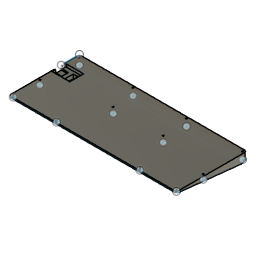
RowLow52V2-bottomcase v4 (Autodesk Fusion 360 design; units mm, degrees)
Autodesk Fusion 360 part; units mm, degrees
sketch "スケッチ1" plane through (0, 0, 0) normal (0, 0, 1) x (1, 0, 0)
  line L0 (239.1777, -2.4183) -> (239.1601, -97.857)
  spline S0 degree 3 poles (239.1601, -97.857) (239.1855, -99.2018) (238.1172, -100.3131) (236.7725, -100.3413) knots 0 0 0 0 1 1 1 1
  line L1 (236.7725, -100.3413) -> (2.6363, -100.3547)
  spline S1 degree 3 poles (2.6363, -100.3547) (1.2915, -100.3801) (0.1799, -99.3119) (0.152, -97.9671) knots 0 0 0 0 1 1 1 1
  line L2 (0.152, -97.9671) -> (0.152, -2.5093)
  spline S2 degree 3 poles (0.152, -2.5093) (0.1266, -1.1645) (1.1949, -0.0529) (2.5393, -0.025) knots 0 0 0 0 1 1 1 1
  line L3 (2.5393, -0.025) -> (236.6931, -0.031)
  spline S3 degree 3 poles (236.6931, -0.031) (238.0382, -0.0053) (239.1498, -1.0739) (239.1777, -2.4183) knots 0 0 0 0 1 1 1 1
  line L4 (1.676, -20.726) -> (1.676, -20.98)
  line L5 (1.676, -20.98) -> (1.676, -40.4107)
  line L6 (1.676, -40.4107) -> (26.695, -40.4107)
  line L7 (26.695, -40.4107) -> (26.695, -20.7257)
  line L8 (26.695, -20.7257) -> (2.311, -20.7257)
  line L9 (2.311, -20.7257) -> (1.676, -20.726)
  line L10 (1.676, -20.726) -> (1.676, -20.98)
  line L11 (10.312, -35.204) -> (10.312, -35.458)
  line L12 (2.692, -26.06) -> (0.025, -26.06)
  line L13 (0.025, -26.06) -> (0.025, -35.458)
  line L14 (0.025, -35.458) -> (10.312, -35.458)
  line L15 (10.312, -35.458) -> (10.312, -35.204)
  line L16 (10.312, -35.204) -> (10.312, -26.06)
  line L17 (10.312, -26.06) -> (2.692, -26.06)
  line L18 (22.123, -37.236) -> (22.123, -24.282)
  line L19 (22.123, -24.282) -> (15.646, -24.282)
  line L20 (15.646, -24.282) -> (15.646, -37.236)
  line L21 (15.646, -37.236) -> (22.123, -37.236)
  circle A0 centre (155.346, -2.311) radius 1.1
  circle A1 centre (236.2447, -3.073) radius 1.1
  circle A2 centre (183.921, -97.561) radius 1.1
  circle A3 centre (2.946, -97.561) radius 1.1
  circle A4 centre (2.946, -59.461) radius 1.1
  circle A5 centre (88.798, -40.411) radius 1.1
  circle A6 centre (64.922, -97.561) radius 1.1
  circle A7 centre (160.172, -40.411) radius 1.1
  circle A8 centre (79.273, -2.565) radius 1.1
  circle A9 centre (236.372, -59.461) radius 1.1
  circle A10 centre (236.2447, -97.561) radius 1.1
  circle A11 centre (2.946, -2.819) radius 1.1
  point P0 (156.446, -2.311)
  point P1 (237.3447, -3.073)
  point P2 (185.021, -97.561)
  point P3 (4.046, -97.561)
  point P4 (4.046, -59.461)
  point P5 (89.898, -40.411)
  point P6 (66.022, -97.561)
  point P7 (161.272, -40.411)
  point P8 (80.373, -2.565)
  point P9 (237.472, -59.461)
  point P10 (237.3447, -97.561)
  point P11 (4.046, -2.819)
extrude "押し出し1" add sketch "スケッチ1" against normal blind 40 contours L0 S0 L1 S1 L2 S2 L3 S3 L4 L5 L6 L7 L8 L9 L10 L12 L14 | L2 L5 L12 L14 | L5 L11 L12 L14 L15 L16 L17 | L4 L5 L6 L7 L8 L9 L10 L11 L12 L14 L15 L16 L17 | L18 L19 L20 L21
extrude "押し出し2" cut sketch "スケッチ1" against normal blind 6 contours L2 L5 L12 L14 | L5 L11 L12 L14 L15 L16 L17
extrude "押し出し3" cut sketch "スケッチ1" against normal blind 4 contours L4 L5 L6 L7 L8 L9 L10 L11 L12 L14 L15 L16 L17
extrude "押し出し4" cut sketch "スケッチ1" against normal blind 40 contours L18 L19 L20 L21
sketch "スケッチ2" plane through (0, 0, 0) normal (1, 0, 0) x (0, 1, 0)
  line L0 (-100.355, 0) -> (-100.355, -2)
  line L1 (-100.355, -2) -> (3, -13)
  line L2 (-7.5019, -11.8823) -> (0.5, -9)
  line L3 (-100.355, -2) -> (-100.57, -2)
  line L4 (-100.57, -2) -> (-100.57, -3.4)
  line L5 (-100.57, -3.4) -> (-100.57, -40.4093)
  line L6 (-100.57, -40.4093) -> (-74, -40.4093)
  line L7 (-74, -40.4093) -> (1, -40.4093)
  line L8 (1, -40.4093) -> (0.5, -9)
  dimension "d9" = 2
  constraint vertical L0
  constraint coincident L1 L2.start
  constraint perpendicular L0 L3
  constraint perpendicular L3 L4
  constraint parallel L4 L5
  constraint perpendicular L5 L6
  constraint parallel L6 L7
  measures "d9" distance of L0.start L0.end
extrude "押し出し5" cut sketch "スケッチ2" along normal blind 400 contours L1 L3 L4 L5 L6 L7 L8
extrude "押し出し6" cut sketch "スケッチ2" along normal blind 400 contours L1 L2 L8
sketch "スケッチ3" plane through (0, 0, 0) normal (1, 0, 0) x (0, 1, 0)
  line L0 (0.1398, 0.1029) -> (-26.06, 0.1029)
  constraint horizontal L0
sketch "スケッチ4" plane through (0, -1.3345, -12.5387) normal (0, -0.105832, -0.994384) x (1, 0, 0)
  ellipse E0 centre (160.172, 39.2973) end of major axis (160.172, 38.1911) minor radius 1.1
  ellipse E1 centre (236.2447, 96.77) end of major axis (236.2447, 95.6638) minor radius 1.1
  ellipse E2 centre (183.921, 96.77) end of major axis (183.921, 95.6638) minor radius 1.1
  ellipse E3 centre (236.372, 58.4548) end of major axis (236.372, 57.3487) minor radius 1.1
  ellipse E4 centre (88.798, 39.2973) end of major axis (88.798, 38.1911) minor radius 1.1
  ellipse E5 centre (2.946, 96.77) end of major axis (2.946, 95.6638) minor radius 1.1
  ellipse E6 centre (2.946, 58.4548) end of major axis (2.946, 57.3487) minor radius 1.1
  ellipse E7 centre (64.922, 96.77) end of major axis (64.922, 95.6638) minor radius 1.1
  line L0 (22.123, 36.1043) -> (22.123, 23.0772)
  line L1 (22.123, 23.0772) -> (15.646, 23.0772)
  line L2 (15.646, 23.0772) -> (15.646, 36.1043)
  line L3 (15.646, 36.1043) -> (22.123, 36.1043)
  line L4 (0.152, 6.2022) -> (239.1768, 6.2022)
  line L5 (239.1768, 6.2022) -> (239.1601, 97.0677)
  spline S0 degree 3 poles (236.7725, 99.566) (236.9396, 99.5624) (237.1056, 99.542) (237.4266, 99.4681) (237.5804, 99.4159) (238.0207, 99.2151) (238.2841, 99.0244) (238.7171, 98.5588) (238.8855, 98.2893) (239.1117, 97.6993) (239.166, 97.3855) (239.1601, 97.0677) knots -0.385662 -0.385662 -0.385662 -0.385662 -0.335417 -0.335417 -0.286659 -0.286659 -0.189937 -0.189937 -0.095378 -0.095378 0 0 0 0
  line L6 (236.7725, 99.566) -> (2.6363, 99.5794)
  spline S1 degree 3 poles (2.6151, 99.5798) (2.6222, 99.5797) (2.6292, 99.5796) (2.6363, 99.5794) knots -0.002119 -0.002119 -0.002119 -0.002119 0 0 0 0
  line L7 (2.6151, 99.5798) -> (2.5636, 99.5798)
  spline S2 degree 3 poles (0.152, 97.1784) (0.1556, 97.3498) (0.1766, 97.52) (0.2528, 97.8488) (0.3067, 98.0062) (0.5108, 98.4494) (0.702, 98.7126) (1.1661, 99.1426) (1.4326, 99.3091) (1.9922, 99.5233) (2.2757, 99.5767) (2.5636, 99.5798) knots -0.385525 -0.385525 -0.385525 -0.385525 -0.334027 -0.334027 -0.284114 -0.284114 -0.187392 -0.187392 -0.093864 -0.093864 -0.00728 -0.00728 -0.00728 -0.00728
  line L8 (0.152, 97.1784) -> (0.152, 6.2022)
  circle A0 centre (2.946, 96.77) radius 2.3941
  circle A1 centre (2.946, 58.4548) radius 2.3046
  circle A2 centre (64.922, 96.77) radius 2.3483
  circle A3 centre (183.921, 96.77) radius 2.2833
  circle A4 centre (236.2447, 96.77) radius 2.2651
  circle A5 centre (236.372, 58.4548) radius 2.3236
  circle A6 centre (160.172, 39.2973) radius 2.3586
  circle A7 centre (88.798, 39.2973) radius 2.4454
  constraint concentric E5 A0
  constraint concentric E6 A1
  constraint concentric E7 A2
  constraint concentric E2 A3
  constraint concentric E1 A4
  constraint concentric E3 A5
  constraint concentric E0 A6
  constraint concentric E4 A7
extrude "押し出し7" cut sketch "スケッチ4" against normal blind 1 contours E5 | A0
extrude "押し出し8" cut sketch "スケッチ4" against normal blind 1 contours E7 | A2
extrude "押し出し9" cut sketch "スケッチ4" against normal blind 1 contours E2 | A3
extrude "押し出し10" cut sketch "スケッチ4" against normal blind 1 contours E1 | A4
extrude "押し出し11" cut sketch "スケッチ4" against normal blind 1.5 contours E6 | A1
extrude "押し出し12" cut sketch "スケッチ4" against normal blind 1.5 contours E4 | A7
extrude "押し出し13" cut sketch "スケッチ4" against normal blind 1.5 contours E0 | A6
extrude "押し出し14" cut sketch "スケッチ4" against normal blind 1.5 contours E3 | A5
sketch "スケッチ5" plane through (0, 2.9269, -8.1258) normal (0, 0.338887, -0.940827) x (-1, 0, 0)
  line L0 (-0.152, -11.0847) -> (-0.152, -5.7781)
  spline S0 degree 3 poles (-2.5393, -3.1376) (-2.3792, -3.1412) (-2.2204, -3.1611) (-1.9125, -3.2329) (-1.7647, -3.2837) (-1.3412, -3.4784) (-1.0881, -3.6623) (-0.6398, -4.1342) (-0.4566, -4.4267) (-0.2063, -5.0743) (-0.1458, -5.4243) (-0.152, -5.7781) knots -0.397498 -0.397498 -0.397498 -0.397498 -0.349267 -0.349267 -0.302241 -0.302241 -0.208829 -0.208829 -0.106159 -0.106159 0 0 0 0
  line L1 (-2.5393, -3.1376) -> (-236.6931, -3.144)
  spline S1 degree 3 poles (-239.1777, -5.6814) (-239.1738, -5.4825) (-239.1489, -5.285) (-239.0577, -4.9055) (-238.9933, -4.7246) (-238.7664, -4.2552) (-238.5683, -3.9872) (-238.1011, -3.5623) (-237.8426, -3.4012) (-237.2827, -3.1885) (-236.9901, -3.138) (-236.6931, -3.144) knots -0.395915 -0.395915 -0.395915 -0.395915 -0.3363 -0.3363 -0.278857 -0.278857 -0.179915 -0.179915 -0.08914 -0.08914 0 0 0 0
  line L2 (-239.1777, -5.6814) -> (-239.1768, -11.0847)
  line L3 (-239.1768, -11.0847) -> (-0.152, -11.0847)
  ellipse E0 centre (-155.346, -5.5674) end of major axis (-155.346, -4.3983) minor radius 1.1
  ellipse E1 centre (-2.946, -6.1074) end of major axis (-2.946, -4.9382) minor radius 1.1
  ellipse E2 centre (-236.2447, -6.3773) end of major axis (-236.2447, -5.2082) minor radius 1.1
  ellipse E3 centre (-79.273, -5.8374) end of major axis (-79.273, -4.6682) minor radius 1.1
  circle A0 centre (-2.946, -6.1074) radius 2.2782
  circle A1 centre (-79.273, -5.8374) radius 2.3234
  circle A2 centre (-155.346, -5.5674) radius 2.2538
  circle A3 centre (-236.2447, -6.3773) radius 2.2901
  constraint concentric E1 A0
  constraint concentric E3 A1
  constraint concentric E0 A2
  constraint concentric E2 A3
extrude "押し出し15" cut sketch "スケッチ5" against normal blind 1.5 contours E1 | A0
extrude "押し出し16" cut sketch "スケッチ5" against normal blind 1.5 contours E3 | A1
extrude "押し出し17" cut sketch "スケッチ5" against normal blind 1.5 contours E0 | A2
extrude "押し出し18" cut sketch "スケッチ5" against normal blind 1.5 contours E2 | A3
